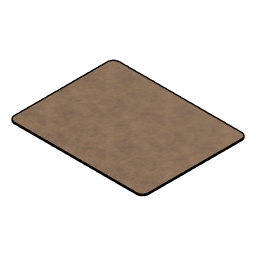
Mousepad-V1 (Autodesk Fusion 360 design; units mm, degrees)
Autodesk Fusion 360 part; units mm, degrees
sketch "Skizze1" plane through (0, 0, 0) normal (0, 0, 1) x (1, 0, 0)
  line L0 (-12.0523, 42.3584) -> (197.9477, 42.3584)
  line L1 (207.9477, 32.3584) -> (207.9477, -127.6416)
  line L2 (197.9477, -137.6416) -> (-12.0523, -137.6416)
  line L3 (-22.0523, -127.6416) -> (-22.0523, 32.3584)
  arc A0 (-12.0523, 42.3584) -> (-22.0523, 32.3584) centre (-12.0523, 32.3584) ccw
  arc A1 (207.9477, 32.3584) -> (197.9477, 42.3584) centre (197.9477, 32.3584) ccw
  arc A2 (197.9477, -137.6416) -> (207.9477, -127.6416) centre (197.9477, -127.6416) ccw
  arc A3 (-22.0523, -127.6416) -> (-12.0523, -137.6416) centre (-12.0523, -127.6416) ccw
  point P0 (-22.0523, 42.3584)
  point P1 (207.9477, 42.3584)
  point P2 (-22.0523, -137.6416)
  dimension "d1" = 230
  dimension "d2" = 180
  dimension "d3" = 10
  constraint horizontal L0
  constraint vertical L1
  constraint horizontal L2
  constraint vertical L3
  constraint coincident P0 L0
  constraint coincident P0 L3
  constraint tangent L0 A0
  constraint tangent L3 A0
  constraint coincident P1 L0
  constraint coincident P1 L1
  constraint tangent L0 A1
  constraint tangent L1 A1
  constraint equal A0 A1
  constraint tangent L1 A2
  constraint tangent L2 A2
  constraint equal A0 A2
  constraint coincident P2 L2
  constraint coincident P2 L3
  constraint tangent L2 A3
  constraint tangent L3 A3
  constraint equal A0 A3
  measures "d1" distance of P0 P1
  measures "d2" distance of P0 P2
  measures "d3" radius of A0
extrude "Extrusion1" add sketch "Skizze1" along normal blind 2
named bodies: "body"
